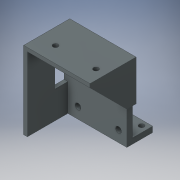
# Autodesk Inventor part: PantatKanan
Saved by Autodesk Inventor 2016 (Build 200138000, 138)
## iProperties
Created: 2017-05-09
Part Number: PantatKanan
Material: Iron, Gray
Document SubType Name: Modeling
Designer: Ghana
Density: 7.15 g/cm^3
Appearance: Iron Gray
Author: Ghana
Autodesk Inventor part; units mm, degrees
ref_plane "YZ Plane" through (0, 0, 0) normal (1, 0, 0) x (0, 1, 0)
ref_plane "XZ Plane" through (0, 0, 0) normal (0, 1, 0) x (-1, 0, 0)
ref_plane "XY Plane" through (0, 0, 0) normal (0, 0, 1) x (1, 0, 0)
sketch "Sketch1" plane through (0, 0, 0) normal (0, 1, 0) x (-1, 0, 0)
  line L0 (0, 0) -> (34, 0)
  line L1 (34, 0) -> (34, -14)
  line L2 (34, -14) -> (0, -14)
  line L3 (0, -14) -> (0, 0)
  dimension "d0" = 34
  dimension "d1" = 14
  constraints: 8 end point, 2 parallel, 1 horizontal, 1 perpendicular
  measures "d0" distance of L1.end L2.end
  measures "d1" distance of L0.end L1.end
extrude "Extrusion1" add sketch "Sketch1" along normal blind 3
sketch "Sketch2" plane through (0, 3, 0) normal (0, 1, 0) x (1, 0, 0)
  line L0 (-34, 0) -> (0, 0) projected
  line L1 (0, 0) -> (0, 14) projected
  line L2 (0, 14) -> (-34, 14) projected
  line L3 (-34, 14) -> (-34, 0) projected
  point P0 (-25.23, 11.2)
  point P1 (-3.23, 11.2)
  dimension "d59" = 22
  dimension "d60" = 8.77
  measures "d59" distance of point (-25.23, 11.2) point (-3.23, 11.2)
  measures "d60" distance from line of L3 point (-25.23, 11.2)
hole "Hole1" at (-25.23, 3, -11.2) at (-3.23, 3, -11.2) direction (0, -1, 0) diameter 2.7 end through all
sketch "Sketch3" plane through (0, 3, 0) normal (0, 1, 0) x (1, 0, 0)
  circle A0 centre (-25.23, 11.2) radius 1.35 projected
  circle A1 centre (-3.23, 11.2) radius 1.35 projected
  line L0 (-34, 0) -> (0, 0) projected
  line L1 (0, 0) -> (0, 14) projected
  line L2 (0, 14) -> (-34, 14) projected
  line L3 (-34, 14) -> (-34, 0) projected
  line L4 (0, 0) -> (-34, 0) projected
  line L5 (-34, 0) -> (0, 0)
  line L6 (0, 0) -> (0, 3)
  line L7 (0, 3) -> (-34, 3)
  line L8 (-34, 3) -> (-34, 0)
  dimension "d14" = 3
  constraints: 8 end point, 2 parallel, 1 horizontal, 1 perpendicular, 1 point on line
  measures "d14" distance of L6.end L5.end
extrude "Extrusion2" add sketch "Sketch3" along normal blind 39 contours L3 L7 L1 L0
sketch "Sketch4" plane through (0, 42, 0) normal (0, 1, 0) x (1, 0, 0)
  line L0 (-34, 0) -> (0, 0) projected
  line L1 (0, 0) -> (0, 3) projected
  line L2 (0, 3) -> (-34, 3) projected
  line L3 (-34, 3) -> (-34, 0) projected
  line L4 (-34, 3) -> (0, 3)
  line L5 (0, 3) -> (0, -22)
  line L6 (0, -22) -> (-34, -22)
  line L7 (-34, -22) -> (-34, 3)
  dimension "d17" = 25
  constraints: 8 end point, 2 parallel, 1 horizontal, 1 perpendicular
  measures "d17" distance of L4.end L5.end
extrude "Extrusion3" add sketch "Sketch4" against normal blind 2 contours L0 L5 L6 L7
sketch "Sketch6" plane through (0, 42, 0) normal (0, 1, 0) x (1, 0, 0)
  line L0 (0, -22) -> (0, 3) projected
  line L1 (0, 3) -> (-34, 3) projected
  line L2 (-34, 3) -> (-34, -22) projected
  line L3 (-34, -22) -> (0, -22) projected
  line L4 (0, 14) -> (0, -22) projected
  point P0 (0, 0)
  point P1 (-3.23, -13.5)
  point P2 (-25.23, -13.5)
  dimension "d57" = 22
  dimension "d58" = 3.23
  measures "d57" distance of point (-3.23, -13.5) point (-25.23, -13.5)
  measures "d58" distance from line of L0 point (-3.23, -13.5)
hole "Hole2" at (-3.23, 42, 13.5) at (-25.23, 42, 13.5) direction (0, -1, 0) diameter 2.7 end through all
sketch "Sketch7" plane through (-34, 0, 0) normal (0, 0, 1) x (1, 0, 0)
  line L0 (34, 40) -> (0, 40) projected
  line L1 (0, 0) -> (0, 40) projected
  line L2 (34, 0) -> (0, 0) projected
  line L3 (34, 0) -> (34, 40) projected
  point P0 (7.5, 6)
  point P1 (29.5, 6)
  point P2 (18.5, 35.5)
  dimension "d50" = 11
  dimension "d51" = 29.5
  dimension "d52" = 22
  dimension "d55" = 4.5
  measures "d50" horizontal distance of point (7.5, 6) point (18.5, 35.5)
  measures "d51" vertical distance of point (7.5, 6) point (18.5, 35.5)
  measures "d52" distance of point (29.5, 6) point (7.5, 6)
  measures "d55" distance from line of L3 point (29.5, 6)
hole "Hole3" at (-26.5, 6, 0) at (-4.5, 6, 0) at (-15.5, 35.5, 0) direction (0, 0, -1) diameter 3.2 end through all
sketch "Sketch8" plane through (-34, 0, 0) normal (0, 0, 1) x (1, 0, 0)
  circle A0 centre (29.5, 6) radius 1.6 projected
  circle A1 centre (7.5, 6) radius 1.6 projected
  circle A2 centre (18.5, 35.5) radius 1.6 projected
  line L0 (34, 40) -> (0, 40) projected
  line L1 (0, 0) -> (0, 40) projected
  line L2 (34, 0) -> (0, 0) projected
  line L3 (14.5, 34.5) -> (4.5, 34.5)
  line L4 (4.5, 34.5) -> (4.5, 26.5)
  line L5 (4.5, 26.5) -> (14.5, 26.5)
  line L6 (14.5, 26.5) -> (14.5, 34.5)
  line L7 (34, 0) -> (34, 40) projected
  dimension "d46" = 10
  dimension "d47" = 8
  dimension "d53" = 1
  dimension "d54" = 4
  constraints: 8 end point, 2 parallel, 1 horizontal, 1 perpendicular
  measures "d46" distance of L5.end L4.end
  measures "d47" distance of L4.end L3.end
  measures "d53" distance from line of L3 A2.centre
  measures "d54" distance from line of L6 A2.centre
extrude "Extrusion5" cut sketch "Sketch8" against normal blind 3 contours L6 L5 L4 L3
sketch "Sketch9" plane through (-34, 0, -14) normal (-1, 0, 0) x (0, 0, 1)
  line L0 (14, 0) -> (0, 0) projected
  line L1 (14, 0) -> (14, 40) projected
  line L2 (36, 40) -> (14, 40) projected
  line L3 (36, 42) -> (36, 40) projected
  line L4 (11, 42) -> (36, 42) projected
  line L5 (11, 3) -> (11, 42) projected
  line L6 (0, 3) -> (11, 3) projected
  line L7 (0, 0) -> (0, 3) projected
  line L8 (14, 40) -> (36, 40)
  line L9 (36, 40) -> (36, 0)
  line L10 (36, 0) -> (14, 0)
  line L11 (14, 0) -> (14, 40)
  constraints: 8 end point, 2 parallel, 1 horizontal, 1 perpendicular
extrude "Extrusion6" add sketch "Sketch9" against normal blind 2 contours L1 L2 L9 L10
sketch "Sketch10" plane through (0, 0, 0) normal (1, 0, 0) x (0, 0, -1)
  line L0 (14, 0) -> (0, 0) projected
  line L1 (14, 0) -> (14, 3) projected
  line L2 (3, 3) -> (14, 3) projected
  line L3 (3, 3) -> (3, 42) projected
  line L4 (-22, 42) -> (3, 42) projected
  line L5 (-22, 42) -> (-22, 40) projected
  line L6 (0, 40) -> (-22, 40) projected
  line L7 (0, 0) -> (0, 40) projected
  line L8 (-22, 42) -> (-22, 40) projected
  line L9 (3, 3) -> (3, 42) projected
  line L10 (-22, 42) -> (3, 42)
  line L11 (3, 42) -> (3, 20)
  line L12 (3, 20) -> (-22, 20)
  line L13 (-22, 20) -> (-22, 42)
  dimension "d63" = 22
  constraints: 8 end point, 2 parallel, 1 horizontal, 1 perpendicular, 1 point on line
  measures "d63" distance of L10.end L11.end
extrude "Extrusion7" add sketch "Sketch10" along normal blind 2 contours L12 L13 L6 L7 | L7 L6 L5 L4 L3 L12
chamfer "Chamfer1" distance 2 angle 45 1 edges at (0, 20, -1.5)
chamfer "Chamfer2" distance 20 angle 45 1 edges at (1, 20, 22)
chamfer "Chamfer3" distance 1.99 angle 45 1 edges at (0.9999, 20, 0)
sketch "Sketch11" plane through (-34, 0, -14) normal (-1, 0, 0) x (0, 0, 1)
  line L0 (14, 40) -> (14, 0) projected
  line L1 (36, 40) -> (14, 40) projected
  line L2 (14, 40) -> (21, 40)
  line L3 (21, 40) -> (21, 15)
  line L4 (21, 15) -> (14, 15)
  line L5 (14, 15) -> (14, 40)
  dimension "d75" = 7
  dimension "d76" = 25
  constraints: 8 end point, 2 parallel, 1 horizontal, 1 perpendicular
  measures "d75" distance of L3.end L4.end
  measures "d76" distance of L2.end L3.end
extrude "Extrusion8" cut sketch "Sketch11" against normal blind 2
sketch "Sketch12" plane through (0, 3, 0) normal (0, 1, 0) x (1, 0, 0)
  line L0 (-34, 3) -> (0, 3) projected
  line L1 (0, 3) -> (0, 14) projected
  line L2 (0, 14) -> (-34, 14) projected
  line L3 (-34, 14) -> (-34, 3) projected
  circle A0 centre (-25.23, 11.2) radius 1.35 projected
  circle A1 centre (-3.23, 11.2) radius 1.35 projected
  line L4 (-34, 3) -> (0, 3) projected
  line L5 (-3.23, 11.2) -> (-8.23, 11.2)
  line L6 (-8.23, 11.2) -> (-8.23, 3)
  line L7 (-8.23, 3) -> (-3.23, 3)
  line L8 (-3.23, 3) -> (-3.23, 11.2)
  line L9 (-25.23, 11.2) -> (-22.23, 11.2)
  line L10 (-22.23, 11.2) -> (-22.23, 3)
  line L11 (-22.23, 3) -> (-25.23, 3)
  line L12 (-25.23, 3) -> (-25.23, 11.2)
  line L13 (-8.23, 3) -> (-22.23, 3)
  line L14 (-22.23, 3) -> (-22.23, 7)
  line L15 (-22.23, 7) -> (-8.23, 7)
  line L16 (-8.23, 7) -> (-8.23, 3)
  point P0 (0, 0)
  dimension "d79" = 5
  dimension "d80" = 3
  dimension "d81" = 4
  constraints: 24 end point, 6 parallel, 3 horizontal, 3 perpendicular, 3 point on line
  measures "d79" distance of L7.end L6.end
  measures "d80" distance of L10.end L11.end
  measures "d81" distance of L13.end L14.end
extrude "Extrusion9" add sketch "Sketch12" along normal blind 7 contours L10 L15 L6 L0
chamfer "Chamfer4" distance 4 angle 45 1 edges at (-15.23, 10, -7)
body "Solid1"
